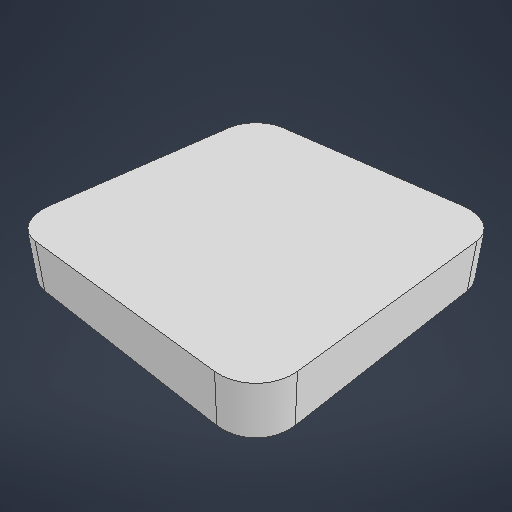
# Autodesk Inventor part: keycap
Saved by Autodesk Inventor 2025.2 (Build 292293000, 293)
## iProperties
Created: 2025-10-01
Part Number: keycap
Material: Generic
Document SubType Name: Modeling
Designer: nebes
Density: 1 g/cm^3
Appearance: Default
Author: nebes
Autodesk Inventor part; units mm, degrees
ref_plane "YZ Plane" through (0, 0, 0) normal (1, 0, 0) x (0, 1, 0)
ref_plane "XZ Plane" through (0, 0, 0) normal (0, 1, 0) x (-1, 0, 0)
ref_plane "XY Plane" through (0, 0, 0) normal (0, 0, 1) x (1, 0, 0)
sketch "Sketch1" plane through (0, 0, 0) normal (0, 1, 0) x (-1, 0, 0)
  line L0 (-8.55, 8.55) -> (8.55, 8.55)
  line L1 (8.55, 8.55) -> (8.55, -8.55)
  line L2 (8.55, -8.55) -> (-8.55, -8.55)
  line L3 (-8.55, -8.55) -> (-8.55, 8.55)
  line L4 (-8.55, 8.55) -> (8.55, -8.55) construction
  line L5 (8.55, 8.55) -> (-8.55, -8.55) construction
  line L6 (7.55, 7.55) -> (-7.55, 7.55)
  line L7 (-7.55, 7.55) -> (-7.55, -7.55)
  line L8 (-7.55, -7.55) -> (7.55, -7.55)
  line L9 (7.55, -7.55) -> (7.55, 7.55)
  line L10 (7.55, 7.55) -> (-7.55, -7.55) construction
  line L11 (-7.55, 7.55) -> (7.55, -7.55) construction
  line L12 (1.5, 2.35) -> (-1.5, 2.35)
  line L13 (-1.5, 2.35) -> (-1.5, 3.35)
  line L14 (-1.5, 3.35) -> (1.5, 3.35)
  line L15 (1.5, 3.35) -> (1.5, 2.35)
  line L16 (1.5, 2.35) -> (-1.5, 3.35) construction
  line L17 (-1.5, 2.35) -> (1.5, 3.35) construction
  line L18 (1.5, -3.35) -> (-1.5, -3.35)
  line L19 (-1.5, -3.35) -> (-1.5, -2.35)
  line L20 (-1.5, -2.35) -> (1.5, -2.35)
  line L21 (1.5, -2.35) -> (1.5, -3.35)
  line L22 (1.5, -3.35) -> (-1.5, -2.35) construction
  line L23 (-1.5, -3.35) -> (1.5, -2.35) construction
  line L24 (0, 0) -> (-1, 0)
  circle A0 centre (-6.3, 6.3) radius 1.25
  circle A1 centre (-6.3, 6.3) radius 2.25
  circle A2 centre (-6.3, -6.3) radius 1.25
  circle A3 centre (-6.3, -6.3) radius 2.25
  circle A4 centre (6.3, -6.3) radius 1.25
  circle A5 centre (6.3, -6.3) radius 2.25
  circle A6 centre (6.3, 6.3) radius 1.25
  circle A7 centre (6.3, 6.3) radius 2.25
  point P0 (0, 2.85)
  point P1 (0, -2.85)
  point P2 (-8.55, 6.3)
  point P3 (-8.55, -6.3)
  point P4 (-6.3, -8.55)
  point P5 (6.3, -8.55)
  point P6 (8.55, -6.3)
  point P7 (8.55, 6.3)
  point P8 (6.3, 8.55)
  point P9 (-6.3, 8.55)
  point P10 (-7.55, 6.3)
  point P11 (-6.3, 7.55)
  point P12 (6.3, 7.55)
  point P13 (7.55, 6.3)
  point P14 (7.55, -6.3)
  point P15 (6.3, -7.55)
  point P16 (-6.3, -7.55)
  point P17 (-7.55, -6.3)
  dimension "d0" = 17.1
  dimension "d1" = 17.1
  dimension "d4" = 1
  dimension "d5" = 1
  dimension "d6" = 5.7
  dimension "d7" = 3
  dimension "d8" = 1
  dimension "d10" = 2.5
  constraints: 50 end point, 12 tangent, 8 centre point, 8 midpoint, 8 parallel, 5 horizontal, 4 coincident, 4 perpendicular, 3 equal radius, 2 equal length, 2 vertical alignment, 1 point on line, 1 other
  measures "d0" distance of L1.end L2.end
  measures "d1" distance of L0.end L1.end
  measures "d4" distance between parallel lines of L2 L8
  measures "d5" distance of L24.start L24.end
  measures "d6" distance of point (0, -2.85) point (0, 2.85)
  measures "d7" distance of L13.end L14.end
  measures "d8" distance of L12.end L13.end
  measures "d10" diameter of A0
extrude "Extrusion2" add sketch "Sketch1" along normal blind 1 contours L0 A7 L6 A1 | A1 L6 L7 | A1 L7 A3 L3 | A7 L9 L6 | A1 L7 A0 L6 | L6 A7 L9 A5 L8 A3 L7 A1 | A3 L7 L8 | L1 A5 L9 A7 | L6 A6 L9 A7 | A0 L7 L6 | A0 | A3 L8 A2 L7 | A3 L8 A5 L2 | A5 L8 L9 | L6 L9 A6 | A6 | A2 L8 L7 | A2 | L9 A4 L8 A5 | A4 | L9 L8 A4 | L12 L13 L14 L15 | L18 L19 L20 L21
extrude "Extrusion3" add sketch "Sketch1" against normal blind 2 contours L0 A7 L6 A1 | A1 L6 L7 | A1 L7 A3 L3 | A7 L9 L6 | A3 L7 L8 | L1 A5 L9 A7 | A0 L7 L6 | A3 L8 A5 L2 | A5 L8 L9 | L6 L9 A6 | A2 L8 L7 | L9 L8 A4
extrude "Extrusion4" add sketch "Sketch1" against normal blind 3 contours L12 L13 L14 L15 | L18 L19 L20 L21
body "Solid2"
